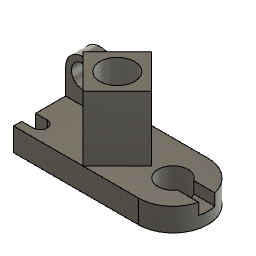
drawing_17 v1 (Autodesk Fusion 360 design; units mm, degrees)
Autodesk Fusion 360 part; units mm, degrees
sketch "Sketch1" plane through (0, 0, 0) normal (0, 1, 0) x (1, 0, 0)
  line L0 (10, -10) -> (118, -10)
  line L1 (148, -40) -> (148, -40)
  line L2 (118, -70) -> (10, -70)
  line L3 (10, -70) -> (10, -10)
  arc A0 (148, -40) -> (118, -10) centre (118, -40) ccw
  arc A1 (118, -70) -> (148, -40) centre (118, -40) ccw
  circle A2 centre (118, -40) radius 13
  point P0 (148, -10)
  dimension "d1" = 138
  dimension "d2" = 60
  dimension "d3" = 30
  dimension "d4" = 30
  dimension "d5" = 26
  constraint horizontal L0
  constraint horizontal L2
  constraint vertical L3
  constraint coincident P0 L0
  constraint tangent L0 A0
  constraint tangent L2 A1
  constraint concentric A0 A2
  measures "d1" distance of L0.start P0
  measures "d2" distance of L0.start L2.end
  measures "d3" radius of A0
  measures "d4" radius of A1
  measures "d5" diameter of A2
extrude "Extrude1" add sketch "Sketch1" along normal blind 20
sketch "Sketch2" plane through (0, 20, 0) normal (0, 1, 0) x (-1, 0, 0)
  circle A0 centre (-118, 40) radius 13
  line L0 (-10, 70) -> (-118, 70)
  arc A1 (-118, 70) -> (-118, 10) centre (-118, 40) ccw
  line L1 (-118, 10) -> (-10, 10)
  line L2 (-10, 10) -> (-10, 70)
  line L3 (-118, 47) -> (-155, 47)
  arc A2 (-155, 47) -> (-155, 33) centre (-155, 40) ccw
  line L4 (-155, 33) -> (-118, 33)
  arc A3 (-118, 33) -> (-118, 47) centre (-118, 40) ccw
  line L5 (-118, 40) -> (-155, 40) construction
  dimension "d8" = 14
  constraint tangent L3 A2
  constraint tangent A2 L4
  constraint parallel L3 L4
  constraint tangent L4 A3
  constraint tangent L3 A3
  constraint parallel L1 L5
  constraint coincident A0.centre A1.centre
  measures "d8" diameter of A2
extrude "Extrude2" cut sketch "Sketch2" against normal blind 10 contours A0 A1 L3 L4
sketch "Sketch4" plane through (0, 20, 0) normal (0, 1, 0) x (-1, 0, 0)
  line L0 (-147.1719, 47) -> (-128.9545, 47)
  arc A0 (-128.9545, 33) -> (-128.9545, 47) centre (-118, 40) ccw
  line L1 (-128.9545, 33) -> (-147.1719, 33)
  arc A1 (-147.1719, 33) -> (-118, 10) centre (-118, 40) ccw
  line L2 (-118, 10) -> (-10, 10)
  line L3 (-10, 10) -> (-10, 70)
  line L4 (-10, 70) -> (-118, 70)
  arc A2 (-118, 70) -> (-147.1719, 47) centre (-118, 40) ccw
  line L5 (-10, 70) -> (-70, 70) construction
  line L6 (-70, 70) -> (-70, 10) construction
  line L7 (-70, 70) -> (-40.3015, 40.3015) construction
  line L8 (-70, 70) -> (-28, 70) construction
  line L9 (-70, 70) -> (-40.3015, 40.3015)
  line L10 (-40.3015, 40.3015) -> (-70, 10.603)
  line L11 (-70, 10.603) -> (-99.6985, 40.3015)
  line L12 (-99.6985, 40.3015) -> (-70, 70)
  dimension "d11" = 60
  dimension "d12" = 45
  dimension "d13" = 42
  dimension "d14" = 42
  constraint coincident L3.end L4.start
  constraint perpendicular L3 L5
  constraint coincident L2 L6.end
  constraint perpendicular L2 L6
  constraint horizontal L8
  constraint perpendicular L9 L10
  constraint parallel L9 L11
  constraint parallel L10 L12
  measures "d11" distance of L3.end L5.end
  measures "d12" angle of L7 L8
  measures "d13" distance of L5.end L7.end
  measures "d14" distance of L5.end L11.end
extrude "Extrude3" add sketch "Sketch4" along normal blind 56 contours L9 L10 L11 L12
hole "Hole1" at (70, 76, 40.3015) direction (0, -1, 0) diameter 30 depth 90 tip angle 180
hole "Hole2" at (70, 0, 40.3015) direction (0, 1, 0) diameter 50 depth 10 tip angle 180
sketch "Sketch5" plane through (0, 20, 0) normal (0, 1, 0) x (-1, 0, 0)
  line L0 (-147.1719, 47) -> (-128.9545, 47)
  arc A0 (-128.9545, 33) -> (-128.9545, 47) centre (-118, 40) ccw
  line L1 (-128.9545, 33) -> (-147.1719, 33)
  arc A1 (-147.1719, 33) -> (-118, 10) centre (-118, 40) ccw
  line L2 (-118, 10) -> (-10, 10)
  line L3 (-10, 10) -> (-10, 70)
  line L4 (-10, 70) -> (-70, 70)
  line L5 (-70, 70) -> (-40.3015, 40.3015)
  line L6 (-40.3015, 40.3015) -> (-70, 10.603)
  line L7 (-70, 10.603) -> (-99.6985, 40.3015)
  line L8 (-99.6985, 40.3015) -> (-70, 70)
  line L9 (-70, 70) -> (-118, 70)
  arc A2 (-118, 70) -> (-147.1719, 47) centre (-118, 40) ccw
  line L10 (-10, 57) -> (-10, 63)
  line L11 (-10, 63) -> (-20, 63)
  line L12 (-20, 51) -> (-10, 51)
  arc A3 (-10, 51) -> (-10, 63) centre (-10, 57) ccw
  line L13 (-10, 63) -> (-20, 63)
  arc A4 (-20, 63) -> (-20, 51) centre (-20, 57) ccw
  line L14 (-20, 57) -> (-10, 57) construction
  dimension "d24" = 6
  dimension "d25" = 10
  constraint parallel L3 L10
  constraint perpendicular L3 L11
  constraint tangent L12 A3
  constraint tangent A3 L13
  constraint parallel L12 L13
  constraint tangent L13 A4
  constraint tangent L12 A4
  constraint coincident L10.start A3.centre
  measures "d24" distance of L10.start L10.end
  measures "d25" distance of L10.end L11.end
extrude "Extrude4" cut sketch "Sketch5" against normal blind 20 contours L3 L10 L11 L12 L13 A4
sketch "Sketch6" plane through (0, 20, 0) normal (0, 1, 0) x (-1, 0, 0)
  line L0 (-20, 63) -> (-10, 63)
  line L1 (-10, 63) -> (-10, 70)
  line L2 (-10, 70) -> (-70, 70)
  line L3 (-70, 70) -> (-40.3015, 40.3015)
  line L4 (-40.3015, 40.3015) -> (-70, 10.603)
  line L5 (-70, 10.603) -> (-99.6985, 40.3015)
  line L6 (-99.6985, 40.3015) -> (-70, 70)
  line L7 (-70, 70) -> (-118, 70)
  arc A0 (-118, 70) -> (-147.1719, 47) centre (-118, 40) ccw
  line L8 (-147.1719, 47) -> (-128.9545, 47)
  arc A1 (-128.9545, 33) -> (-128.9545, 47) centre (-118, 40) ccw
  line L9 (-128.9545, 33) -> (-147.1719, 33)
  arc A2 (-147.1719, 33) -> (-118, 10) centre (-118, 40) ccw
  line L10 (-118, 10) -> (-10, 10)
  line L11 (-10, 10) -> (-10, 51)
  line L12 (-10, 51) -> (-20, 51)
  arc A3 (-20, 63) -> (-20, 51) centre (-20, 57) ccw
  line L13 (-10, 10) -> (-40, 10)
  line L14 (-40, 10) -> (-40, 25)
  line L15 (-40, 25) -> (-10, 25)
  line L16 (-10, 25) -> (-10, 10)
  dimension "d28" = 30
  dimension "d29" = 15
  constraint horizontal L13
  constraint vertical L14
  constraint horizontal L15
  constraint vertical L16
  constraint coincident L10.end L11.start
  measures "d28" distance of L10.end L13.end
  measures "d29" distance of L10.end L15.end
extrude "Extrude5" add sketch "Sketch6" along normal blind 37 contours L10 L11 L13 L14 L15 L16
fillet "Fillet1" radius 15 2 edges at (10, 57, 17.5) (40, 57, 17.5)
hole "Hole3" at (25, 42, 25) direction (0, 0, -1) diameter 20 depth 130 tip angle 180
